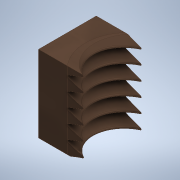
# Autodesk Inventor part: Plaqueta Fosforbronce
Saved by Autodesk Inventor 2020 (Build 240168000, 168)
## iProperties
Created: 2020-09-17
Part Number: Plaqueta Fosforbronce
Material: Bronze
Document SubType Name: Modeling
Designer: aaron
Density: 8.47 g/cm^3
Appearance: Bronze - Satin Hammered
Author: aaron
Autodesk Inventor part; units mm, degrees
ref_plane "YZ Plane" through (0, 0, 0) normal (1, 0, 0) x (0, 1, 0)
ref_plane "XZ Plane" through (0, 0, 0) normal (0, 1, 0) x (-1, 0, 0)
ref_plane "XY Plane" through (0, 0, 0) normal (0, 0, 1) x (1, 0, 0)
sketch "Sketch2" plane through (0, 0, 0) normal (0, 1, 0) x (-1, 0, 0)
  circle A0 centre (0, 0) radius 17.4625
  dimension "d6" = 34.925
  constraints: 2 coincident, 1 centre point
  measures "d6" diameter of A0
extrude "Extrusion2" add sketch "Sketch2" against normal blind 12.7
hole "Hole1" at (0, 0, 0) direction (0, -1, 0) diameter 14.351 end through all thread size "5/8-18 UNF" class "2B" standard "ANSI Unified Screw Threads"
thread "Thread1" size "5/8-11 UNC" class "2B" standard "ANSI Unified Screw Threads" full length
sketch "Sketch5" plane through (0, 0, 0) normal (1, 0, 0) x (0, 0, 1)
  line L0 (7.1755, 0) -> (7.1755, 12.7)
  line L1 (7.1755, 12.7) -> (5.4634, 12.7)
  line L2 (5.4634, 12.7) -> (5.4634, 0)
  line L3 (5.4634, 0) -> (7.1755, 0)
  line L4 (0, -5.5615) -> (0, 15.7436) projected
  constraints: 8 end point
revolve "Revolution1" add sketch "Sketch5" angle 360 about axis through (0, 0, 0) along (0, -1, 0) separate body
sketch "Sketch4" plane through (0, 0, 7.1755) normal (-1, 0, 0) x (0, -1, 0)
  line L0 (-1.3471, -0.1169) -> (-1.1546, -0.1169) construction
  line L1 (0.1923, -1.5955) -> (-0.0001, -1.9652) construction
  line L2 (-2.3092, -1.9652) -> (-2.5016, -1.5955) construction
  line L3 (-0.9622, -0.1169) -> (-1.1546, 0.2527) construction
  line L4 (-1.1546, 0.2527) -> (-1.3471, -0.1169) construction
  line L5 (-2.3092, -1.9652) -> (-2.1168, -1.5955) construction
  line L6 (-0.9622, -0.1169) -> (-0.1925, -1.5955)
  line L7 (-2.5016, -1.5955) -> (-2.1168, -1.5955) construction
  arc A0 (-2.5016, -1.5955) -> (-2.3092, -1.7123) centre (-2.3092, -1.4953) ccw construction
  line L8 (0.1923, -1.5955) -> (-0.1925, -1.5955) construction
  line L9 (-2.3092, -1.9652) -> (-2.3092, -1.5955) construction
  line L10 (-0.0001, -1.9652) -> (-0.0001, -1.5955) construction
  line L11 (-1.1546, 0.2527) -> (-1.1546, -0.0002) construction
  line L12 (-2.3092, -1.7123) -> (-0.0001, -1.7123)
  arc A1 (-2.3092, -1.7123) -> (-2.1168, -1.5955) centre (-2.3092, -1.4953) ccw
  line L13 (-0.1925, -1.5955) -> (-0.0001, -1.9652) construction
  line L14 (-2.1168, -1.5955) -> (-1.3471, -0.1169)
  line L15 (-0.0001, -0.0002) -> (-0.0001, 0.0177)
  line L16 (-0.0001, 0.0177) -> (-0.0001, -0.0002)
  line L17 (-0.0001, -0.0002) -> (0.0334, -0.0002)
  arc A2 (-0.1925, -1.5955) -> (-0.0001, -1.7123) centre (-0.0001, -1.4953) ccw
  arc A3 (-0.0001, -1.7123) -> (0.1923, -1.5955) centre (-0.0001, -1.4953) ccw construction
  arc A4 (-1.1546, -0.0002) -> (-1.3471, -0.1169) centre (-1.1546, -0.2171) ccw
  arc A5 (-0.9622, -0.1169) -> (-1.1546, -0.0002) centre (-1.1546, -0.2171) ccw
  line L18 (-1.1546, -0.0002) -> (-1.1546, -0.1169) construction
  line L19 (-1.1546, -0.1169) -> (-0.9622, -0.1169) construction
  dimension "d22" = 55
  dimension "d23" = 0.3696
  dimension "d24" = 0.3696
  dimension "Sketch4_ThreadOffset" = 0
  dimension "Sketch4_MajorRadius" = 1.7121
  dimension "d27" = 2.3091
  dimension "Sketch4_MinorRadius" = 0
  constraints: 40 end point, 12 point on circle, 10 parallel, 8 tangent, 6 centre point, 6 collinear, 2 midpoint, 2 point on line, 1 horizontal, 1 perpendicular, 3 other
  measures "d22" angle of L6 L14
  measures "d23" distance of L3.end L0.end
  measures "d24" distance of L1.end L10.end
  measures "Sketch4_ThreadOffset" distance between parallel lines of L15 L10
  measures "Sketch4_MajorRadius" distance from line of L12 L15.start
  measures "d27" distance from line of L1.end L9
  measures "Sketch4_MinorRadius" distance edge to line of A5 L17
coil "Coil1" sketch "Sketch4" operation cut axis through (0, 0, 0) along (0, -1, 0) pitch 2.3114 turns 7.492507 hand right bodies 2
sketch "Sketch3" plane through (0, 0, 0) normal (0, 1, 0) x (1, 0, 0)
  circle A0 centre (0, 0) radius 7.1755 projected
  circle A1 centre (0, 0) radius 7.1755 projected
  circle A2 centre (0, 0) radius 17.4625 projected
  line L0 (-24.4475, 0) -> (24.4475, 0) construction
  line L1 (-5.3672, -4.7625) -> (-10.1297, -4.7625)
  line L2 (-10.1297, -4.7625) -> (-10.1297, 0)
  line L3 (-5.3672, 4.7625) -> (-10.1297, 4.7625)
  line L4 (-10.1297, 4.7625) -> (-10.1297, 0)
  line L5 (-5.3672, 4.7625) -> (0, 4.7625)
  line L6 (0, 4.7625) -> (0, -4.7625)
  line L7 (0, -4.7625) -> (-5.3672, -4.7625)
  dimension "d16" = 4.7625
  dimension "d17" = 4.7625
  constraints: 14 end point, 3 perpendicular, 2 horizontal, 2 symmetric about line, 1 point on line, 2 other
  measures "d16" distance of L1.end L2.end
  measures "d17" distance of L1.start L1.end
extrude "Extrusion4" cut sketch "Sketch3" against normal blind 12.7 contours L5 L6 L7 A0 | A0 L1 L2 L4 L3 keep common part picked at (-2.3918, 0) bodies 1 2
equation "\"d22\" = d29"
equation "\"d23\" = 0.160083 * Sketch4_Pitch"
equation "\"d24\" = 0.160083 * Sketch4_Pitch"
equation "\"d27\" = Sketch4_Pitch"
equation "\"d29\" = 55deg"
equation "\"Sketch4_Pitch\" = 2.30909"
body "Solid2"
body "Solid3"
